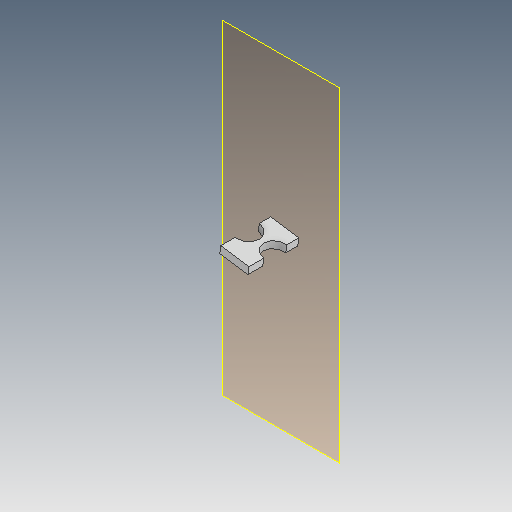
# Autodesk Inventor part: motor mount center
Saved by Autodesk Inventor 2020 (Build 240168000, 168)
## iProperties
Created: 2019-10-21
Part Number: motor mount center
Material: Generic
Document SubType Name: Modeling
Designer: ball
Density: 1 g/cm^3
Appearance: Default
Author: ball
Autodesk Inventor part; units mm, degrees
ref_plane "YZ Plane" through (0, 0, 0) normal (1, 0, 0) x (0, 1, 0)
ref_plane "XZ Plane" through (0, 0, 0) normal (0, 1, 0) x (-1, 0, 0)
ref_plane "Work Plane1" through (0, 0, 0) normal (0, 0, 1) x (1, 0, 0)
sketch "Sketch1" plane through (0, 0, 0) normal (0, 0, 1) x (1, 0, 0)
  line L0 (46.9411, 24.4056) -> (43.9673, 4.6279) construction
  line L1 (-34.7264, 28.3648) -> (-39.7819, -5.2572) construction
  line L2 (9.0191, -106.7418) -> (35.6521, 70.3833) construction
  line L3 (-3.8449, 105.9638) -> (-30.4779, -71.1613) construction
  line L4 (8.3675, 9.9808) -> (26.1674, 7.3043)
  line L5 (8.3675, 9.9808) -> (-17.688, 13.8986)
  line L6 (2.8511, 22.7146) -> (27.9178, 18.9455)
  line L7 (2.8511, 22.7146) -> (-15.9376, 25.5397)
  line L8 (-15.9376, 25.5397) -> (-17.688, 13.8986)
  line L9 (27.9178, 18.9455) -> (26.1674, 7.3043)
  point P0 (0, 0)
  constraints: 20 end point, 4 point on line, 2 collinear, 2 perpendicular, 14 other
ref_plane "Work Plane2" through (-150.8486, -254.8124, 77.677) normal (0, 0, -1) x (0, 1, 0)
extrude "Extrusion1" add sketch "Sketch1" along normal up to surface (77.677 mm away)
sketch "Sketch2" plane through (27.9178, 18.9455, 77.677) normal (0.1487, 0.9889, 0) x (0.9889, -0.1487, 0)
  circle A0 centre (0, 41.0877) radius 18 construction
  circle A1 centre (-44.3484, 41.0877) radius 19 construction
  circle A2 centre (-44.3484, 41.0877) radius 19
  circle A3 centre (0, 41.0877) radius 18
  point P0 (-24.7904, 77.677)
  constraints: 2 centre point, 2 coincident, 2 concentric
extrude "Extrusion2" cut sketch "Sketch2" against normal through all
body "Solid1"
